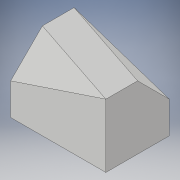
# Autodesk Inventor part: 零件14
Saved by Autodesk Inventor 2019 (Build 230136000, 136)
## iProperties
Created: 2020-09-18
Part Number: 零件14
Material: 一般
Document SubType Name: Modeling
Designer: jay
Density: 1 g/cm^3
Appearance: 預設
Author: jay
Autodesk Inventor part; units mm, degrees
ref_plane "YZ Plane" through (0, 0, 0) normal (1, 0, 0) x (0, 1, 0)
sketch "草圖1" plane through (0, 0, 0) normal (0, 0, 1) x (1, 0, 0)
  line L0 (-12, 0) -> (72, 0) projected
  line L1 (0, -8) -> (0, 48) projected
  line L2 (0, 0) -> (60, 0)
  line L3 (60, 0) -> (60, 40)
  line L4 (60, 40) -> (0, 40)
  line L5 (0, 40) -> (0, 0)
  dimension "d0" = 60
  dimension "d1" = 40
  constraints: 8 end point, 2 parallel, 1 horizontal, 1 perpendicular
  measures "d0" distance of L3.end L4.end
  measures "d1" distance of L2.end L3.end
extrude "擠出1" add sketch "草圖1" along normal blind 40
ref_plane "工作平面1" through (0, 40, 20) normal (-0.2294, 0.6882, 0.6882) x (0, -0.7071, 0.7071)
sketch "草圖2" plane through (0, 40, 20) normal (-0.2294, 0.6882, 0.6882) x (0, -0.7071, 0.7071)
  line L0 (42.4264, 55.1553) -> (14.1421, 61.6441) projected
  line L1 (14.1421, 3.2444) -> (42.4264, -3.2444) projected
  line L2 (-14.1421, -3.2444) -> (14.1421, 3.2444) projected
  line L3 (-24.1266, -29.4243) -> (37.1709, -29.4243)
  line L4 (37.1709, -29.4243) -> (37.1709, 87.3992)
  line L5 (37.1709, 87.3992) -> (-24.1266, 87.3992)
  line L6 (-24.1266, 87.3992) -> (-24.1266, -29.4243)
  point P0 (14.1421, -9.7333)
  constraints: 8 end point, 2 parallel, 1 horizontal, 1 perpendicular
extrude "擠出2" cut sketch "草圖2" along normal blind 40
ref_plane "工作平面3" through (0, 40, 0) normal (0.2294, 0.6882, -0.6882) x (0.9487, 0, 0.3162)
sketch "草圖4" plane through (0, 40, 0) normal (0.2294, 0.6882, -0.6882) x (0.9487, 0, 0.3162)
  line L0 (-18.5971, -44.6398) -> (132.4913, -44.6398)
  line L1 (132.4913, -44.6398) -> (132.4913, 100.0809)
  line L2 (132.4913, 100.0809) -> (-18.5971, 100.0809)
  line L3 (-18.5971, 100.0809) -> (-18.5971, -44.6398)
  point P0 (0, 29.0191)
  constraints: 8 end point, 2 parallel, 1 horizontal, 1 perpendicular
extrude "擠出4" cut sketch "草圖4" along normal blind 40
